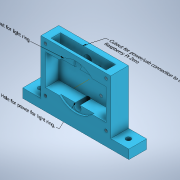
# Autodesk Inventor part: 2020PiZeroCameraLightRingMount
Saved by Autodesk Inventor 2020.2 (Build 242310000, 310)
## iProperties
Created: 2019-10-10
Part Number: 2020PiZeroCameraLightRingMount
Material: PC/ABS Plastic
Document SubType Name: Modeling
Designer: steele
Density: 0.357273 g/cm^3
Appearance: Turquoise
Author: steele
Autodesk Inventor part; units mm, degrees
ref_plane "YZ Plane" through (0, 0, 0) normal (1, 0, 0) x (0, 1, 0)
ref_plane "XZ Plane" through (0, 0, 0) normal (0, 1, 0) x (-1, 0, 0)
ref_plane "XY Plane" through (0, 0, 0) normal (0, 0, 1) x (1, 0, 0)
sketch "Sketch1" plane through (0, 0, 0) normal (0, 0, 1) x (1, 0, 0)
  line L0 (-48.5775, -37.85) -> (48.5775, -37.85)
  line L1 (48.5775, -37.85) -> (48.5775, 37.85)
  line L2 (48.5775, 37.85) -> (-48.5775, 37.85)
  line L3 (-48.5775, 37.85) -> (-48.5775, -37.85)
  line L4 (-48.5775, -37.85) -> (48.5775, 37.85) construction
  line L5 (48.5775, -37.85) -> (-48.5775, 37.85) construction
  point P0 (0, 0)
  dimension "majorPartWidth" = 97.155
  dimension "majorPartHeight" = 75.7
  constraints: 12 end point, 2 midpoint, 2 parallel, 1 horizontal, 1 perpendicular
  measures "majorPartWidth" distance of L0.start L0.end
  measures "majorPartHeight" distance of L1.end L0.end
extrude "Extrusion1" add sketch "Sketch1" against normal blind 24.725
sketch "Sketch2" plane through (0, 0, 0) normal (0, 0, 1) x (1, 0, 0)
  line L0 (-42.2275, -21.59) -> (42.2275, -21.59)
  line L1 (42.2275, -21.59) -> (42.2275, 21.59)
  line L2 (42.2275, 21.59) -> (-42.2275, 21.59)
  line L3 (-42.2275, 21.59) -> (-42.2275, -21.59)
  line L4 (-42.2275, -21.59) -> (42.2275, 21.59) construction
  line L5 (42.2275, -21.59) -> (-42.2275, 21.59) construction
  point P0 (0, 0)
  dimension "holeForPiCaseWidth" = 84.455
  dimension "holeForPiCaseHeight" = 43.18
  constraints: 12 end point, 2 midpoint, 2 parallel, 1 horizontal, 1 perpendicular
  measures "holeForPiCaseWidth" distance of L0.start L0.end
  measures "holeForPiCaseHeight" distance of L1.end L0.end
extrude "Extrusion2" cut sketch "Sketch2" against normal blind 18.375
sketch "Sketch3" plane through (0, 0, 0) normal (0, 0, 1) x (1, 0, 0)
  circle A0 centre (0, 0) radius 31.5
  circle A1 centre (0, 0) radius 18.5
  dimension "lightRingHoleExteriorDiam" = 63
  dimension "lightRingHoleInteriorDiam" = 37
  constraints: 2 centre point, 2 coincident
  measures "lightRingHoleExteriorDiam" diameter of A0
  measures "lightRingHoleInteriorDiam" diameter of A1
extrude "Extrusion3" cut sketch "Sketch3" against normal blind 2.5
sketch "Sketch4" plane through (0, 0, -2.5) normal (0, 0, 1) x (1, 0, 0)
  circle A0 centre (0, 0) radius 25.4466 construction
  circle A1 centre (0, 25.4466) radius 5
  circle A2 centre (0, -25.4466) radius 5
  dimension "holeForLightRingWires" = 10
  dimension "d13" = 10
  constraints: 3 centre point, 2 point on circle, 1 coincident
  measures "holeForLightRingWires" diameter of A1
  measures "d13" diameter of A2
extrude "Extrusion4" cut sketch "Sketch4" against normal through all
sketch "Sketch6" plane through (-48.5775, -37.85, 0) normal (0, -1, 0) x (1, 0, 0)
  line L0 (0, -24.725) -> (97.155, -24.725) projected
  line L1 (0, -24.725) -> (97.155, -24.725)
  line L2 (97.155, -24.725) -> (97.155, 0)
  line L3 (97.155, 0) -> (0, 0)
  line L4 (0, 0) -> (0, -24.725)
  point P0 (48.5775, 0)
  dimension "baseWidth" = 97.155
  dimension "baseDepth" = 24.725
  constraints: 8 end point, 2 parallel, 1 horizontal, 1 perpendicular
  measures "baseWidth" distance of L2.end L3.end
  measures "baseDepth" distance of L1.end L2.end
extrude "Extrusion6" add sketch "Sketch6" along normal blind 12.7
sketch "Sketch7" plane through (-48.5775, 37.85, 0) normal (0, 1, 0) x (1, 0, 0)
  line L0 (97.155, 0) -> (0, 0) construction
  line L1 (0, 0) -> (0, 24.725) construction
  line L2 (10.16, 3.77) -> (86.995, 3.77)
  line L3 (86.995, 3.77) -> (86.995, 17.105)
  line L4 (86.995, 17.105) -> (10.16, 17.105)
  line L5 (10.16, 17.105) -> (10.16, 3.77)
  line L6 (10.16, 3.77) -> (86.995, 17.105) construction
  line L7 (86.995, 3.77) -> (10.16, 17.105) construction
  line L8 (45.3952, 18.375) -> (45.3952, 2.5) projected
  point P0 (48.5775, 0)
  point P1 (48.5775, 10.4375)
  dimension "y" = 10.4375
  dimension "Y" = 48.5775
  dimension "piWireDepth" = 13.335
  dimension "piWireWidth" = 76.835
  constraints: 12 end point, 2 midpoint, 2 parallel, 2 perpendicular
  measures "y" distance from line of point (48.577, 10.438) L0
  measures "Y" distance from line of point (48.577, 10.438) L1
  measures "piWireDepth" distance of L4.end L2.start
  measures "piWireWidth" distance of L3.end L4.end
extrude "Extrusion7" cut sketch "Sketch7" against normal up to next
sketch "Sketch8" plane through (-48.5775, 37.85, -24.725) normal (-1, 0, 0) x (0, 0, 1)
  line L0 (24.725, -75.7) -> (24.725, 0) projected
  line L1 (24.725, -75.7) -> (28.535, -75.7)
  line L2 (28.535, -75.7) -> (28.535, -78.24)
  line L3 (28.535, -78.24) -> (24.725, -78.24)
  line L4 (24.725, -78.24) -> (24.725, -75.7)
  point P0 (24.725, -37.85)
  dimension "d30" = 3.81
  dimension "d31" = 2.54
  constraints: 8 end point, 2 parallel, 1 horizontal, 1 perpendicular
  measures "d30" distance of L2.end L3.end
  measures "d31" distance of L1.end L2.end
extrude "Extrusion8" cut sketch "Sketch8" against normal through all
sketch "Sketch9" plane through (0, 0, 0) normal (0, 0, 1) x (1, 0, 0)
  point P0 (-42.2275, 31.5)
  point P1 (42.2275, 31.5)
  point P2 (42.2275, -31.5)
  point P3 (-42.2275, -31.5)
hole "Hole1" at (-42.2275, 31.5, 0) at (42.2275, 31.5, 0) at (42.2275, -31.5, 0) at (-42.2275, -31.5, 0) direction (0, 0, -1) diameter 3.9624 depth 14.986 tip angle 120 thread size "10-32 UNF" class "2B" standard "ANSI Unified Screw Threads"
sketch "Sketch10" plane through (0, 0, -24.725) normal (0, 0, -1) x (-1, 0, 0)
  point P0 (-39.0525, 23.7022)
  point P1 (-16.8275, 23.7022)
  point P2 (-16.8275, -11.2228)
  point P3 (-39.0525, -11.2228)
hole "Hole3" at (39.0525, 23.7022, -24.725) at (16.8275, 23.7022, -24.725) at (16.8275, -11.2228, -24.725) at (39.0525, -11.2228, -24.725) direction (0, 0, 1) diameter 3.9624 depth 11.9507 tip angle 120 thread size "10-32 UNF" class "2B" standard "ANSI Unified Screw Threads"
sketch "Sketch14" plane through (-48.5775, -50.55, 0) normal (0, -1, 0) x (1, 0, 0)
  circle A0 centre (-12.7, 0) radius 2.5527 construction
  circle A1 centre (109.855, 0) radius 2.5527 construction
  line L0 (-12.7, 0) -> (109.855, 0) construction
  spline S0 degree 2 poles (34.1258, -3.8141) (34.1258, -4.5098) (33.5619, -5.6296) (33.0884, -5.9424) knots 0 0 0 1 2 2 2
  spline S1 degree 2 poles (33.0884, -5.9424) (32.7015, -6.1853) (31.9069, -6.35) (31.2894, -6.35) knots 0 0 0 1 2 2 2
  line L1 (31.2894, -6.35) -> (30.1203, -6.35)
  line L2 (30.1203, -6.35) -> (30.1203, -1.27)
  line L3 (30.1203, -1.27) -> (31.2771, -1.27)
  spline S2 degree 2 poles (31.2771, -1.27) (31.9934, -1.27) (32.8085, -1.4841) (33.0967, -1.6734) knots 0 0 0 1 2 2 2
  spline S3 degree 2 poles (33.0967, -1.6734) (33.5866, -1.9987) (34.1258, -3.0731) (34.1258, -3.8141) knots 0 0 0 1 2 2 2
  spline S4 degree 2 poles (33.4219, -3.8059) (33.4219, -3.2213) (33.0349, -2.3939) (32.6521, -2.1592) knots 0 0 0 1 2 2 2
  spline S5 degree 2 poles (32.6521, -2.1592) (32.3804, -1.9987) (31.767, -1.8546) (31.31, -1.8546) knots 0 0 0 1 2 2 2
  line L4 (31.31, -1.8546) -> (30.7954, -1.8546)
  line L5 (30.7954, -1.8546) -> (30.7954, -5.7654)
  line L6 (30.7954, -5.7654) -> (31.31, -5.7654)
  spline S6 degree 2 poles (31.31, -5.7654) (31.7587, -5.7654) (32.438, -5.6213) (32.7138, -5.4279) knots 0 0 0 1 2 2 2
  spline S7 degree 2 poles (32.7138, -5.4279) (33.0679, -5.1891) (33.4219, -4.3987) (33.4219, -3.8059) knots 0 0 0 1 2 2 2
  spline S8 degree 2 poles (36.4641, -6.4365) (35.5502, -6.4365) (34.5457, -5.4114) (34.5457, -4.4646) knots 0 0 0 1 2 2 2
  spline S9 degree 2 poles (34.5457, -4.4646) (34.5457, -3.5342) (35.5214, -2.4309) (36.3077, -2.4309) knots 0 0 0 1 2 2 2
  spline S10 degree 2 poles (36.3077, -2.4309) (36.6617, -2.4309) (37.2093, -2.6367) (37.411, -2.8549) knots 0 0 0 1 2 2 2
  spline S11 degree 2 poles (37.411, -2.8549) (37.6168, -3.0731) (37.835, -3.703) (37.835, -4.1599) knots 0 0 0 1 2 2 2
  line L7 (37.835, -4.1599) -> (37.835, -4.5098)
  line L8 (37.835, -4.5098) -> (35.1962, -4.5098)
  spline S12 degree 2 poles (35.1962, -4.5098) (35.1962, -5.1726) (35.8631, -5.8766) (36.4559, -5.8766) knots 0 0 0 1 2 2 2
  spline S13 degree 2 poles (36.4559, -5.8766) (36.6658, -5.8766) (37.0734, -5.7819) (37.2381, -5.7078) knots 0 0 0 1 2 2 2
  spline S14 degree 2 poles (37.2381, -5.7078) (37.411, -5.6255) (37.6497, -5.4814) (37.728, -5.4155) knots 0 0 0 1 2 2 2
  line L9 (37.728, -5.4155) -> (37.765, -5.4155)
  line L10 (37.765, -5.4155) -> (37.765, -6.1153)
  spline S15 degree 2 poles (37.765, -6.1153) (37.6539, -6.1606) (37.3163, -6.2924) (37.1846, -6.3294) knots 0 0 0 1 2 2 2
  spline S16 degree 2 poles (37.1846, -6.3294) (36.9993, -6.3829) (36.6947, -6.4365) (36.4641, -6.4365) knots 0 0 0 1 2 2 2
  spline S17 degree 2 poles (37.2093, -4.02) (37.201, -3.7606) (37.094, -3.3819) (36.9911, -3.2542) knots 0 0 0 1 2 2 2
  spline S18 degree 2 poles (36.9911, -3.2542) (36.8799, -3.1102) (36.53, -2.9578) (36.2706, -2.9578) knots 0 0 0 1 2 2 2
  spline S19 degree 2 poles (36.2706, -2.9578) (36.0154, -2.9578) (35.6573, -3.1102) (35.5091, -3.2584) knots 0 0 0 1 2 2 2
  spline S20 degree 2 poles (35.5091, -3.2584) (35.365, -3.4107) (35.2168, -3.7771) (35.1962, -4.02) knots 0 0 0 1 2 2 2
  line L11 (35.1962, -4.02) -> (37.2093, -4.02)
  spline S21 degree 2 poles (39.5146, -6.4406) (39.1317, -6.4406) (38.469, -6.2347) (38.2508, -6.1195) knots 0 0 0 1 2 2 2
  line L12 (38.2508, -6.1195) -> (38.2508, -5.399)
  line L13 (38.2508, -5.399) -> (38.2837, -5.399)
  spline S22 degree 2 poles (38.2837, -5.399) (38.366, -5.4649) (38.5883, -5.6213) (38.7736, -5.7078) knots 0 0 0 1 2 2 2
  spline S23 degree 2 poles (38.7736, -5.7078) (38.9341, -5.786) (39.3293, -5.9013) (39.5393, -5.9013) knots 0 0 0 1 2 2 2
  spline S24 degree 2 poles (39.5393, -5.9013) (39.6916, -5.9013) (40.0415, -5.8313) (40.1239, -5.7737) knots 0 0 0 1 2 2 2
  spline S25 degree 2 poles (40.1239, -5.7737) (40.2433, -5.6954) (40.3503, -5.5184) (40.3503, -5.3373) knots 0 0 0 1 2 2 2
  spline S26 degree 2 poles (40.3503, -5.3373) (40.3503, -5.1109) (40.1033, -4.8762) (39.7863, -4.798) knots 0 0 0 1 2 2 2
  spline S27 degree 2 poles (39.7863, -4.798) (39.6628, -4.7692) (39.2676, -4.6869) (39.0988, -4.6416) knots 0 0 0 1 2 2 2
  spline S28 degree 2 poles (39.0988, -4.6416) (38.6624, -4.514) (38.2672, -3.987) (38.2672, -3.6124) knots 0 0 0 1 2 2 2
  spline S29 degree 2 poles (38.2672, -3.6124) (38.2672, -3.0937) (39.0453, -2.4474) (39.6875, -2.4474) knots 0 0 0 1 2 2 2
  spline S30 degree 2 poles (39.6875, -2.4474) (40.0045, -2.4474) (40.6467, -2.6038) (40.8649, -2.7232) knots 0 0 0 1 2 2 2
  line L14 (40.8649, -2.7232) -> (40.8649, -3.4107)
  line L15 (40.8649, -3.4107) -> (40.8319, -3.4107)
  spline S31 degree 2 poles (40.8319, -3.4107) (40.5849, -3.2131) (39.9839, -2.9867) (39.6752, -2.9867) knots 0 0 0 1 2 2 2
  spline S32 degree 2 poles (39.6752, -2.9867) (39.3582, -2.9867) (38.9218, -3.2542) (38.9218, -3.5218) knots 0 0 0 1 2 2 2
  spline S33 degree 2 poles (38.9218, -3.5218) (38.9218, -3.7647) (39.1811, -3.9994) (39.4693, -4.0735) knots 0 0 0 1 2 2 2
  spline S34 degree 2 poles (39.4693, -4.0735) (39.6093, -4.1105) (39.9633, -4.1846) (40.1568, -4.2299) knots 0 0 0 1 2 2 2
  spline S35 degree 2 poles (40.1568, -4.2299) (40.5767, -4.3369) (41.0048, -4.8268) (41.0048, -5.2508) knots 0 0 0 1 2 2 2
  spline S36 degree 2 poles (41.0048, -5.2508) (41.0048, -5.4978) (40.8114, -5.9342) (40.622, -6.0948) knots 0 0 0 1 2 2 2
  spline S37 degree 2 poles (40.622, -6.0948) (40.4203, -6.2635) (39.9057, -6.4406) (39.5146, -6.4406) knots 0 0 0 1 2 2 2
  line L16 (42.2563, -6.35) -> (41.6141, -6.35)
  line L17 (41.6141, -6.35) -> (41.6141, -2.5379)
  line L18 (41.6141, -2.5379) -> (42.2563, -2.5379)
  line L19 (42.2563, -2.5379) -> (42.2563, -6.35)
  line L20 (42.3016, -1.904) -> (41.5729, -1.904)
  line L21 (41.5729, -1.904) -> (41.5729, -1.2371)
  line L22 (41.5729, -1.2371) -> (42.3016, -1.2371)
  line L23 (42.3016, -1.2371) -> (42.3016, -1.904)
  spline S38 degree 2 poles (43.3349, -6.9593) (43.4008, -6.9881) (43.6519, -7.0787) (43.8124, -7.1157) knots 0 0 0 1 2 2 2
  spline S39 degree 2 poles (43.8124, -7.1157) (43.9894, -7.161) (44.29, -7.2145) (44.467, -7.2145) knots 0 0 0 1 2 2 2
  spline S40 degree 2 poles (44.467, -7.2145) (44.7634, -7.2145) (45.1751, -7.0581) (45.2903, -6.9181) knots 0 0 0 1 2 2 2
  spline S41 degree 2 poles (45.2903, -6.9181) (45.4015, -6.7781) (45.4879, -6.4118) (45.4879, -6.1771) knots 0 0 0 1 2 2 2
  line L24 (45.4879, -6.1771) -> (45.4879, -5.8436)
  spline S42 degree 2 poles (45.4879, -5.8436) (45.2286, -6.0701) (44.7304, -6.2841) (44.3558, -6.2841) knots 0 0 0 1 2 2 2
  spline S43 degree 2 poles (44.3558, -6.2841) (43.7054, -6.2841) (42.9356, -5.3167) (42.9356, -4.4069) knots 0 0 0 1 2 2 2
  spline S44 degree 2 poles (42.9356, -4.4069) (42.9356, -3.9335) (43.2032, -3.2007) (43.4255, -2.9414) knots 0 0 0 1 2 2 2
  spline S45 degree 2 poles (43.4255, -2.9414) (43.6395, -2.6985) (44.2282, -2.4309) (44.5411, -2.4309) knots 0 0 0 1 2 2 2
  spline S46 degree 2 poles (44.5411, -2.4309) (44.8375, -2.4309) (45.2697, -2.5709) (45.4879, -2.6985) knots 0 0 0 1 2 2 2
  line L25 (45.4879, -2.6985) -> (45.525, -2.5379)
  line L26 (45.525, -2.5379) -> (46.1301, -2.5379)
  line L27 (46.1301, -2.5379) -> (46.1301, -5.9136)
  spline S47 degree 2 poles (46.1301, -5.9136) (46.1301, -6.8852) (45.2862, -7.7908) (44.4176, -7.7908) knots 0 0 0 1 2 2 2
  spline S48 degree 2 poles (44.4176, -7.7908) (44.1376, -7.7908) (43.5531, -7.7003) (43.302, -7.6262) knots 0 0 0 1 2 2 2
  line L28 (43.302, -7.6262) -> (43.302, -6.9593)
  line L29 (43.302, -6.9593) -> (43.3349, -6.9593)
  line L30 (45.4879, -5.3167) -> (45.4879, -3.2213)
  spline S49 degree 2 poles (45.4879, -3.2213) (45.2492, -3.106) (44.8457, -3.0072) (44.644, -3.0072) knots 0 0 0 1 2 2 2
  spline S50 degree 2 poles (44.644, -3.0072) (44.1582, -3.0072) (43.5984, -3.7235) (43.5984, -4.3946) knots 0 0 0 1 2 2 2
  spline S51 degree 2 poles (43.5984, -4.3946) (43.5984, -5.0285) (44.0224, -5.6913) (44.4999, -5.6913) knots 0 0 0 1 2 2 2
  spline S52 degree 2 poles (44.4999, -5.6913) (44.751, -5.6913) (45.278, -5.4937) (45.4879, -5.3167) knots 0 0 0 1 2 2 2
  line L31 (50.0533, -6.35) -> (49.4111, -6.35)
  line L32 (49.4111, -6.35) -> (49.4111, -4.1764)
  spline S53 degree 2 poles (49.4111, -4.1764) (49.4111, -3.9129) (49.3617, -3.4601) (49.2876, -3.3242) knots 0 0 0 1 2 2 2
  spline S54 degree 2 poles (49.2876, -3.3242) (49.2094, -3.1801) (48.9295, -3.0402) (48.6907, -3.0402) knots 0 0 0 1 2 2 2
  spline S55 degree 2 poles (48.6907, -3.0402) (48.4519, -3.0402) (47.9456, -3.2954) (47.7027, -3.5012) knots 0 0 0 1 2 2 2
  line L33 (47.7027, -3.5012) -> (47.7027, -6.35)
  line L34 (47.7027, -6.35) -> (47.0605, -6.35)
  line L35 (47.0605, -6.35) -> (47.0605, -2.5379)
  line L36 (47.0605, -2.5379) -> (47.7027, -2.5379)
  line L37 (47.7027, -2.5379) -> (47.7027, -2.962)
  spline S56 degree 2 poles (47.7027, -2.962) (47.9909, -2.7026) (48.5466, -2.4309) (48.8595, -2.4309) knots 0 0 0 1 2 2 2
  spline S57 degree 2 poles (48.8595, -2.4309) (49.4194, -2.4309) (50.0533, -3.1719) (50.0533, -3.8759) knots 0 0 0 1 2 2 2
  line L38 (50.0533, -3.8759) -> (50.0533, -6.35)
  spline S58 degree 2 poles (52.6098, -6.4365) (51.6959, -6.4365) (50.6914, -5.4114) (50.6914, -4.4646) knots 0 0 0 1 2 2 2
  spline S59 degree 2 poles (50.6914, -4.4646) (50.6914, -3.5342) (51.6671, -2.4309) (52.4534, -2.4309) knots 0 0 0 1 2 2 2
  spline S60 degree 2 poles (52.4534, -2.4309) (52.8074, -2.4309) (53.3549, -2.6367) (53.5566, -2.8549) knots 0 0 0 1 2 2 2
  spline S61 degree 2 poles (53.5566, -2.8549) (53.7625, -3.0731) (53.9807, -3.703) (53.9807, -4.1599) knots 0 0 0 1 2 2 2
  line L39 (53.9807, -4.1599) -> (53.9807, -4.5098)
  line L40 (53.9807, -4.5098) -> (51.3419, -4.5098)
  spline S62 degree 2 poles (51.3419, -4.5098) (51.3419, -5.1726) (52.0088, -5.8766) (52.6016, -5.8766) knots 0 0 0 1 2 2 2
  spline S63 degree 2 poles (52.6016, -5.8766) (52.8115, -5.8766) (53.2191, -5.7819) (53.3837, -5.7078) knots 0 0 0 1 2 2 2
  spline S64 degree 2 poles (53.3837, -5.7078) (53.5566, -5.6255) (53.7954, -5.4814) (53.8736, -5.4155) knots 0 0 0 1 2 2 2
  line L41 (53.8736, -5.4155) -> (53.9107, -5.4155)
  line L42 (53.9107, -5.4155) -> (53.9107, -6.1153)
  spline S65 degree 2 poles (53.9107, -6.1153) (53.7995, -6.1606) (53.462, -6.2924) (53.3302, -6.3294) knots 0 0 0 1 2 2 2
  spline S66 degree 2 poles (53.3302, -6.3294) (53.145, -6.3829) (52.8403, -6.4365) (52.6098, -6.4365) knots 0 0 0 1 2 2 2
  spline S67 degree 2 poles (53.3549, -4.02) (53.3467, -3.7606) (53.2397, -3.3819) (53.1367, -3.2542) knots 0 0 0 1 2 2 2
  spline S68 degree 2 poles (53.1367, -3.2542) (53.0256, -3.1102) (52.6757, -2.9578) (52.4163, -2.9578) knots 0 0 0 1 2 2 2
  spline S69 degree 2 poles (52.4163, -2.9578) (52.1611, -2.9578) (51.8029, -3.1102) (51.6547, -3.2584) knots 0 0 0 1 2 2 2
  spline S70 degree 2 poles (51.6547, -3.2584) (51.5106, -3.4107) (51.3624, -3.7771) (51.3419, -4.02) knots 0 0 0 1 2 2 2
  line L43 (51.3419, -4.02) -> (53.3549, -4.02)
  line L44 (57.5622, -6.35) -> (56.92, -6.35)
  line L45 (56.92, -6.35) -> (56.92, -5.963)
  spline S71 degree 2 poles (56.92, -5.963) (56.7718, -6.0865) (56.5536, -6.2512) (56.4054, -6.3212) knots 0 0 0 1 2 2 2
  spline S72 degree 2 poles (56.4054, -6.3212) (56.2695, -6.3871) (55.9773, -6.457) (55.7838, -6.457) knots 0 0 0 1 2 2 2
  spline S73 degree 2 poles (55.7838, -6.457) (55.4709, -6.457) (54.944, -6.1977) (54.7587, -5.9466) knots 0 0 0 1 2 2 2
  spline S74 degree 2 poles (54.7587, -5.9466) (54.5735, -5.6954) (54.3676, -4.9544) (54.3676, -4.4728) knots 0 0 0 1 2 2 2
  spline S75 degree 2 poles (54.3676, -4.4728) (54.3676, -3.9706) (54.627, -3.2378) (54.8534, -2.962) knots 0 0 0 1 2 2 2
  spline S76 degree 2 poles (54.8534, -2.962) (55.0634, -2.715) (55.652, -2.4309) (55.9773, -2.4309) knots 0 0 0 1 2 2 2
  spline S77 degree 2 poles (55.9773, -2.4309) (56.2613, -2.4309) (56.6853, -2.5585) (56.92, -2.6903) knots 0 0 0 1 2 2 2
  line L46 (56.92, -2.6903) -> (56.92, -1.0436)
  line L47 (56.92, -1.0436) -> (57.5622, -1.0436)
  line L48 (57.5622, -1.0436) -> (57.5622, -6.35)
  line L49 (56.92, -5.4237) -> (56.92, -3.2213)
  spline S78 degree 2 poles (56.92, -3.2213) (56.6812, -3.106) (56.3025, -3.0196) (56.0843, -3.0196) knots 0 0 0 1 2 2 2
  spline S79 degree 2 poles (56.0843, -3.0196) (55.5903, -3.0196) (55.0304, -3.7606) (55.0304, -4.4604) knots 0 0 0 1 2 2 2
  spline S80 degree 2 poles (55.0304, -4.4604) (55.0304, -5.1356) (55.4586, -5.8478) (55.932, -5.8478) knots 0 0 0 1 2 2 2
  spline S81 degree 2 poles (55.932, -5.8478) (56.1831, -5.8478) (56.6936, -5.6172) (56.92, -5.4237) knots 0 0 0 1 2 2 2
  spline S82 degree 2 poles (63.869, -4.3822) (63.869, -5.3167) (62.9633, -6.457) (62.2799, -6.457) knots 0 0 0 1 2 2 2
  spline S83 degree 2 poles (62.2799, -6.457) (61.9712, -6.457) (61.5307, -6.3047) (61.3166, -6.173) knots 0 0 0 1 2 2 2
  line L50 (61.3166, -6.173) -> (61.2754, -6.35)
  line L51 (61.2754, -6.35) -> (60.6744, -6.35)
  line L52 (60.6744, -6.35) -> (60.6744, -1.0436)
  line L53 (60.6744, -1.0436) -> (61.3166, -1.0436)
  line L54 (61.3166, -1.0436) -> (61.3166, -2.9373)
  spline S84 degree 2 poles (61.3166, -2.9373) (61.5595, -2.7191) (62.1235, -2.4309) (62.4816, -2.4309) knots 0 0 0 1 2 2 2
  spline S85 degree 2 poles (62.4816, -2.4309) (63.128, -2.4309) (63.869, -3.4642) (63.869, -4.3822) knots 0 0 0 1 2 2 2
  spline S86 degree 2 poles (63.2062, -4.4316) (63.2062, -3.7482) (62.7904, -3.0402) (62.3293, -3.0402) knots 0 0 0 1 2 2 2
  spline S87 degree 2 poles (62.3293, -3.0402) (62.07, -3.0402) (61.5348, -3.2872) (61.3166, -3.4765) knots 0 0 0 1 2 2 2
  line L55 (61.3166, -3.4765) -> (61.3166, -5.6625)
  spline S88 degree 2 poles (61.3166, -5.6625) (61.5595, -5.7819) (61.9341, -5.8807) (62.1564, -5.8807) knots 0 0 0 1 2 2 2
  spline S89 degree 2 poles (62.1564, -5.8807) (62.6463, -5.8807) (63.2062, -5.185) (63.2062, -4.4316) knots 0 0 0 1 2 2 2
  line L56 (67.5287, -2.5379) -> (65.4786, -7.7538)
  line L57 (65.4786, -7.7538) -> (64.7911, -7.7538)
  line L58 (64.7911, -7.7538) -> (65.4745, -6.1647)
  line L59 (65.4745, -6.1647) -> (64.0913, -2.5379)
  line L60 (64.0913, -2.5379) -> (64.7829, -2.5379)
  line L61 (64.7829, -2.5379) -> (65.8244, -5.362)
  line L62 (65.8244, -5.362) -> (66.8618, -2.5379)
  line L63 (66.8618, -2.5379) -> (67.5287, -2.5379)
  line L64 (36.5115, -14.8583) -> (35.6346, -14.8583)
  line L65 (35.6346, -14.8583) -> (34.0291, -12.837)
  line L66 (34.0291, -12.837) -> (33.2552, -12.837)
  line L67 (33.2552, -12.837) -> (33.2552, -14.8583)
  line L68 (33.2552, -14.8583) -> (32.58, -14.8583)
  line L69 (32.58, -14.8583) -> (32.58, -9.7783)
  line L70 (32.58, -9.7783) -> (33.8891, -9.7783)
  spline S90 degree 2 poles (33.8891, -9.7783) (34.3255, -9.7783) (34.9142, -9.873) (35.1818, -10.0459) knots 0 0 0 1 2 2 2
  spline S91 degree 2 poles (35.1818, -10.0459) (35.4494, -10.2188) (35.7581, -10.7581) (35.7581, -11.1574) knots 0 0 0 1 2 2 2
  spline S92 degree 2 poles (35.7581, -11.1574) (35.7581, -11.7131) (35.19, -12.4665) (34.7042, -12.6476) knots 0 0 0 1 2 2 2
  line L71 (34.7042, -12.6476) -> (36.5115, -14.8583)
  spline S93 degree 2 poles (35.0542, -11.2109) (35.0542, -10.9886) (34.8977, -10.6469) (34.7331, -10.5358) knots 0 0 0 1 2 2 2
  spline S94 degree 2 poles (34.7331, -10.5358) (34.589, -10.4411) (34.2061, -10.3629) (33.9262, -10.3629) knots 0 0 0 1 2 2 2
  line L72 (33.9262, -10.3629) -> (33.2552, -10.3629)
  line L73 (33.2552, -10.3629) -> (33.2552, -12.273)
  line L74 (33.2552, -12.273) -> (33.848, -12.273)
  spline S95 degree 2 poles (33.848, -12.273) (34.1403, -12.273) (34.6054, -12.1701) (34.766, -12.0095) knots 0 0 0 1 2 2 2
  spline S96 degree 2 poles (34.766, -12.0095) (34.9142, -11.8696) (35.0542, -11.4744) (35.0542, -11.2109) knots 0 0 0 1 2 2 2
  spline S97 degree 2 poles (39.9983, -12.9523) (39.9983, -13.9156) (39.0721, -14.9653) (38.2981, -14.9653) knots 0 0 0 1 2 2 2
  spline S98 degree 2 poles (38.2981, -14.9653) (37.5036, -14.9653) (36.5938, -13.8826) (36.5938, -12.9523) knots 0 0 0 1 2 2 2
  spline S99 degree 2 poles (36.5938, -12.9523) (36.5938, -11.9972) (37.5324, -10.9392) (38.2981, -10.9392) knots 0 0 0 1 2 2 2
  spline S100 degree 2 poles (38.2981, -10.9392) (39.0721, -10.9392) (39.9983, -11.9931) (39.9983, -12.9523) knots 0 0 0 1 2 2 2
  spline S101 degree 2 poles (39.3355, -12.9523) (39.3355, -12.2113) (38.7962, -11.4908) (38.2981, -11.4908) knots 0 0 0 1 2 2 2
  spline S102 degree 2 poles (38.2981, -11.4908) (37.8, -11.4908) (37.2566, -12.2113) (37.2566, -12.9523) knots 0 0 0 1 2 2 2
  spline S103 degree 2 poles (37.2566, -12.9523) (37.2566, -13.6727) (37.8, -14.4137) (38.2981, -14.4137) knots 0 0 0 1 2 2 2
  spline S104 degree 2 poles (38.2981, -14.4137) (38.7921, -14.4137) (39.3355, -13.685) (39.3355, -12.9523) knots 0 0 0 1 2 2 2
  spline S105 degree 2 poles (43.8515, -12.8905) (43.8515, -13.825) (42.9459, -14.9653) (42.2625, -14.9653) knots 0 0 0 1 2 2 2
  spline S106 degree 2 poles (42.2625, -14.9653) (41.9537, -14.9653) (41.5133, -14.813) (41.2992, -14.6813) knots 0 0 0 1 2 2 2
  line L75 (41.2992, -14.6813) -> (41.258, -14.8583)
  line L76 (41.258, -14.8583) -> (40.657, -14.8583)
  line L77 (40.657, -14.8583) -> (40.657, -9.5519)
  line L78 (40.657, -9.5519) -> (41.2992, -9.5519)
  line L79 (41.2992, -9.5519) -> (41.2992, -11.4455)
  spline S107 degree 2 poles (41.2992, -11.4455) (41.5421, -11.2274) (42.1061, -10.9392) (42.4642, -10.9392) knots 0 0 0 1 2 2 2
  spline S108 degree 2 poles (42.4642, -10.9392) (43.1105, -10.9392) (43.8515, -11.9725) (43.8515, -12.8905) knots 0 0 0 1 2 2 2
  spline S109 degree 2 poles (43.1887, -12.9399) (43.1887, -12.2565) (42.773, -11.5485) (42.3119, -11.5485) knots 0 0 0 1 2 2 2
  spline S110 degree 2 poles (42.3119, -11.5485) (42.0525, -11.5485) (41.5174, -11.7955) (41.2992, -11.9848) knots 0 0 0 1 2 2 2
  line L80 (41.2992, -11.9848) -> (41.2992, -14.1708)
  spline S111 degree 2 poles (41.2992, -14.1708) (41.5421, -14.2902) (41.9167, -14.389) (42.139, -14.389) knots 0 0 0 1 2 2 2
  spline S112 degree 2 poles (42.139, -14.389) (42.6289, -14.389) (43.1887, -13.6933) (43.1887, -12.9399) knots 0 0 0 1 2 2 2
  spline S113 degree 2 poles (48.1658, -14.9489) (47.6142, -14.9489) (46.8403, -14.7183) (46.4986, -14.5537) knots 0 0 0 1 2 2 2
  line L81 (46.4986, -14.5537) -> (46.4986, -13.7056)
  line L82 (46.4986, -13.7056) -> (46.548, -13.7056)
  spline S114 degree 2 poles (46.548, -13.7056) (46.8814, -14.0185) (47.7253, -14.3643) (48.1164, -14.3643) knots 0 0 0 1 2 2 2
  spline S115 degree 2 poles (48.1164, -14.3643) (48.6763, -14.3643) (49.2485, -13.8991) (49.2485, -13.5162) knots 0 0 0 1 2 2 2
  spline S116 degree 2 poles (49.2485, -13.5162) (49.2485, -13.2116) (48.948, -12.8329) (48.6228, -12.7382) knots 0 0 0 1 2 2 2
  spline S117 degree 2 poles (48.6228, -12.7382) (48.3881, -12.6723) (47.997, -12.5818) (47.7048, -12.5077) knots 0 0 0 1 2 2 2
  spline S118 degree 2 poles (47.7048, -12.5077) (47.4413, -12.4377) (47.0255, -12.2277) (46.865, -12.0589) knots 0 0 0 1 2 2 2
  spline S119 degree 2 poles (46.865, -12.0589) (46.7085, -11.8902) (46.5356, -11.4373) (46.5356, -11.1409) knots 0 0 0 1 2 2 2
  spline S120 degree 2 poles (46.5356, -11.1409) (46.5356, -10.5234) (47.4989, -9.6877) (48.244, -9.6877) knots 0 0 0 1 2 2 2
  spline S121 degree 2 poles (48.244, -9.6877) (48.6722, -9.6877) (49.4297, -9.8565) (49.7549, -10.0171) knots 0 0 0 1 2 2 2
  line L83 (49.7549, -10.0171) -> (49.7549, -10.8239)
  line L84 (49.7549, -10.8239) -> (49.7055, -10.8239)
  spline S122 degree 2 poles (49.7055, -10.8239) (49.4626, -10.6016) (48.7051, -10.2723) (48.2893, -10.2723) knots 0 0 0 1 2 2 2
  spline S123 degree 2 poles (48.2893, -10.2723) (47.82, -10.2723) (47.2396, -10.7128) (47.2396, -11.0709) knots 0 0 0 1 2 2 2
  spline S124 degree 2 poles (47.2396, -11.0709) (47.2396, -11.392) (47.5813, -11.7749) (47.9024, -11.8613) knots 0 0 0 1 2 2 2
  spline S125 degree 2 poles (47.9024, -11.8613) (48.1164, -11.919) (48.7381, -12.0672) (48.9439, -12.1289) knots 0 0 0 1 2 2 2
  spline S126 degree 2 poles (48.9439, -12.1289) (49.4667, -12.2895) (49.9525, -12.9358) (49.9525, -13.4092) knots 0 0 0 1 2 2 2
  spline S127 degree 2 poles (49.9525, -13.4092) (49.9525, -13.7097) (49.7096, -14.2861) (49.4914, -14.4878) knots 0 0 0 1 2 2 2
  spline S128 degree 2 poles (49.4914, -14.4878) (49.2485, -14.7101) (48.631, -14.9489) (48.1658, -14.9489) knots 0 0 0 1 2 2 2
  spline S129 degree 2 poles (51.7432, -14.9324) (51.2204, -14.9324) (50.6317, -14.3355) (50.6317, -13.6891) knots 0 0 0 1 2 2 2
  line L85 (50.6317, -13.6891) -> (50.6317, -11.5773)
  line L86 (50.6317, -11.5773) -> (50.1995, -11.5773)
  line L87 (50.1995, -11.5773) -> (50.1995, -11.0462)
  line L88 (50.1995, -11.0462) -> (50.6317, -11.0462)
  line L89 (50.6317, -11.0462) -> (50.6317, -9.9512)
  line L90 (50.6317, -9.9512) -> (51.2739, -9.9512)
  line L91 (51.2739, -9.9512) -> (51.2739, -11.0462)
  line L92 (51.2739, -11.0462) -> (52.4554, -11.0462)
  line L93 (52.4554, -11.0462) -> (52.4554, -11.5773)
  line L94 (52.4554, -11.5773) -> (51.2739, -11.5773)
  line L95 (51.2739, -11.5773) -> (51.2739, -13.3927)
  spline S130 degree 2 poles (51.2739, -13.3927) (51.2739, -13.6809) (51.2945, -13.9979) (51.3645, -14.1338) knots 0 0 0 1 2 2 2
  spline S131 degree 2 poles (51.3645, -14.1338) (51.4221, -14.2531) (51.6815, -14.3725) (51.9038, -14.3725) knots 0 0 0 1 2 2 2
  spline S132 degree 2 poles (51.9038, -14.3725) (52.0602, -14.3725) (52.3525, -14.2778) (52.4184, -14.249) knots 0 0 0 1 2 2 2
  line L96 (52.4184, -14.249) -> (52.4554, -14.249)
  line L97 (52.4554, -14.249) -> (52.4554, -14.8254)
  spline S133 degree 2 poles (52.4554, -14.8254) (52.2743, -14.8748) (51.9038, -14.9324) (51.7432, -14.9324) knots 0 0 0 1 2 2 2
  spline S134 degree 2 poles (54.5838, -14.9447) (53.6698, -14.9447) (52.6654, -13.9197) (52.6654, -12.9728) knots 0 0 0 1 2 2 2
  spline S135 degree 2 poles (52.6654, -12.9728) (52.6654, -12.0425) (53.641, -10.9392) (54.4273, -10.9392) knots 0 0 0 1 2 2 2
  spline S136 degree 2 poles (54.4273, -10.9392) (54.7814, -10.9392) (55.3289, -11.145) (55.5306, -11.3632) knots 0 0 0 1 2 2 2
  spline S137 degree 2 poles (55.5306, -11.3632) (55.7364, -11.5814) (55.9546, -12.2113) (55.9546, -12.6682) knots 0 0 0 1 2 2 2
  line L98 (55.9546, -12.6682) -> (55.9546, -13.0181)
  line L99 (55.9546, -13.0181) -> (53.3158, -13.0181)
  spline S138 degree 2 poles (53.3158, -13.0181) (53.3158, -13.6809) (53.9827, -14.3849) (54.5755, -14.3849) knots 0 0 0 1 2 2 2
  spline S139 degree 2 poles (54.5755, -14.3849) (54.7855, -14.3849) (55.193, -14.2902) (55.3577, -14.2161) knots 0 0 0 1 2 2 2
  spline S140 degree 2 poles (55.3577, -14.2161) (55.5306, -14.1338) (55.7694, -13.9897) (55.8476, -13.9238) knots 0 0 0 1 2 2 2
  line L100 (55.8476, -13.9238) -> (55.8846, -13.9238)
  line L101 (55.8846, -13.9238) -> (55.8846, -14.6236)
  spline S141 degree 2 poles (55.8846, -14.6236) (55.7735, -14.6689) (55.4359, -14.8007) (55.3042, -14.8377) knots 0 0 0 1 2 2 2
  spline S142 degree 2 poles (55.3042, -14.8377) (55.1189, -14.8912) (54.8143, -14.9447) (54.5838, -14.9447) knots 0 0 0 1 2 2 2
  spline S143 degree 2 poles (55.3289, -12.5282) (55.3206, -12.2689) (55.2136, -11.8902) (55.1107, -11.7625) knots 0 0 0 1 2 2 2
  spline S144 degree 2 poles (55.1107, -11.7625) (54.9995, -11.6185) (54.6496, -11.4661) (54.3903, -11.4661) knots 0 0 0 1 2 2 2
  spline S145 degree 2 poles (54.3903, -11.4661) (54.135, -11.4661) (53.7769, -11.6185) (53.6287, -11.7667) knots 0 0 0 1 2 2 2
  spline S146 degree 2 poles (53.6287, -11.7667) (53.4846, -11.919) (53.3364, -12.2854) (53.3158, -12.5282) knots 0 0 0 1 2 2 2
  line L102 (53.3158, -12.5282) -> (55.3289, -12.5282)
  spline S147 degree 2 poles (58.26, -14.9447) (57.3461, -14.9447) (56.3416, -13.9197) (56.3416, -12.9728) knots 0 0 0 1 2 2 2
  spline S148 degree 2 poles (56.3416, -12.9728) (56.3416, -12.0425) (57.3172, -10.9392) (58.1035, -10.9392) knots 0 0 0 1 2 2 2
  spline S149 degree 2 poles (58.1035, -10.9392) (58.4576, -10.9392) (59.0051, -11.145) (59.2068, -11.3632) knots 0 0 0 1 2 2 2
  spline S150 degree 2 poles (59.2068, -11.3632) (59.4126, -11.5814) (59.6308, -12.2113) (59.6308, -12.6682) knots 0 0 0 1 2 2 2
  line L103 (59.6308, -12.6682) -> (59.6308, -13.0181)
  line L104 (59.6308, -13.0181) -> (56.992, -13.0181)
  spline S151 degree 2 poles (56.992, -13.0181) (56.992, -13.6809) (57.6589, -14.3849) (58.2517, -14.3849) knots 0 0 0 1 2 2 2
  spline S152 degree 2 poles (58.2517, -14.3849) (58.4617, -14.3849) (58.8692, -14.2902) (59.0339, -14.2161) knots 0 0 0 1 2 2 2
  spline S153 degree 2 poles (59.0339, -14.2161) (59.2068, -14.1338) (59.4456, -13.9897) (59.5238, -13.9238) knots 0 0 0 1 2 2 2
  line L105 (59.5238, -13.9238) -> (59.5608, -13.9238)
  line L106 (59.5608, -13.9238) -> (59.5608, -14.6236)
  spline S154 degree 2 poles (59.5608, -14.6236) (59.4497, -14.6689) (59.1121, -14.8007) (58.9804, -14.8377) knots 0 0 0 1 2 2 2
  spline S155 degree 2 poles (58.9804, -14.8377) (58.7951, -14.8912) (58.4905, -14.9447) (58.26, -14.9447) knots 0 0 0 1 2 2 2
  spline S156 degree 2 poles (59.0051, -12.5282) (58.9969, -12.2689) (58.8898, -11.8902) (58.7869, -11.7625) knots 0 0 0 1 2 2 2
  spline S157 degree 2 poles (58.7869, -11.7625) (58.6757, -11.6185) (58.3258, -11.4661) (58.0665, -11.4661) knots 0 0 0 1 2 2 2
  spline S158 degree 2 poles (58.0665, -11.4661) (57.8112, -11.4661) (57.4531, -11.6185) (57.3049, -11.7667) knots 0 0 0 1 2 2 2
  spline S159 degree 2 poles (57.3049, -11.7667) (57.1608, -11.919) (57.0126, -12.2854) (56.992, -12.5282) knots 0 0 0 1 2 2 2
  line L107 (56.992, -12.5282) -> (59.0051, -12.5282)
  line L108 (60.9358, -14.8583) -> (60.2936, -14.8583)
  line L109 (60.2936, -14.8583) -> (60.2936, -9.5519)
  line L110 (60.2936, -9.5519) -> (60.9358, -9.5519)
  line L111 (60.9358, -9.5519) -> (60.9358, -14.8583)
  spline S160 degree 2 poles (63.5334, -14.9447) (62.6195, -14.9447) (61.6151, -13.9197) (61.6151, -12.9728) knots 0 0 0 1 2 2 2
  spline S161 degree 2 poles (61.6151, -12.9728) (61.6151, -12.0425) (62.5907, -10.9392) (63.377, -10.9392) knots 0 0 0 1 2 2 2
  spline S162 degree 2 poles (63.377, -10.9392) (63.731, -10.9392) (64.2786, -11.145) (64.4803, -11.3632) knots 0 0 0 1 2 2 2
  spline S163 degree 2 poles (64.4803, -11.3632) (64.6861, -11.5814) (64.9043, -12.2113) (64.9043, -12.6682) knots 0 0 0 1 2 2 2
  line L112 (64.9043, -12.6682) -> (64.9043, -13.0181)
  line L113 (64.9043, -13.0181) -> (62.2655, -13.0181)
  spline S164 degree 2 poles (62.2655, -13.0181) (62.2655, -13.6809) (62.9324, -14.3849) (63.5252, -14.3849) knots 0 0 0 1 2 2 2
  spline S165 degree 2 poles (63.5252, -14.3849) (63.7352, -14.3849) (64.1427, -14.2902) (64.3074, -14.2161) knots 0 0 0 1 2 2 2
  spline S166 degree 2 poles (64.3074, -14.2161) (64.4803, -14.1338) (64.7191, -13.9897) (64.7973, -13.9238) knots 0 0 0 1 2 2 2
  line L114 (64.7973, -13.9238) -> (64.8343, -13.9238)
  line L115 (64.8343, -13.9238) -> (64.8343, -14.6236)
  spline S167 degree 2 poles (64.8343, -14.6236) (64.7232, -14.6689) (64.3856, -14.8007) (64.2539, -14.8377) knots 0 0 0 1 2 2 2
  spline S168 degree 2 poles (64.2539, -14.8377) (64.0686, -14.8912) (63.764, -14.9447) (63.5334, -14.9447) knots 0 0 0 1 2 2 2
  spline S169 degree 2 poles (64.2786, -12.5282) (64.2703, -12.2689) (64.1633, -11.8902) (64.0604, -11.7625) knots 0 0 0 1 2 2 2
  spline S170 degree 2 poles (64.0604, -11.7625) (63.9492, -11.6185) (63.5993, -11.4661) (63.34, -11.4661) knots 0 0 0 1 2 2 2
  spline S171 degree 2 poles (63.34, -11.4661) (63.0847, -11.4661) (62.7266, -11.6185) (62.5784, -11.7667) knots 0 0 0 1 2 2 2
  spline S172 degree 2 poles (62.5784, -11.7667) (62.4343, -11.919) (62.2861, -12.2854) (62.2655, -12.5282) knots 0 0 0 1 2 2 2
  line L116 (62.2655, -12.5282) -> (64.2786, -12.5282)
  line L117 (46.8794, -18.1672) -> (45.1298, -23.2472)
  line L118 (45.1298, -23.2472) -> (44.4011, -23.2472)
  line L119 (44.4011, -23.2472) -> (42.6515, -18.1672)
  line L120 (42.6515, -18.1672) -> (43.3761, -18.1672)
  line L121 (43.3761, -18.1672) -> (44.784, -22.3868)
  line L122 (44.784, -22.3868) -> (46.1919, -18.1672)
  line L123 (46.1919, -18.1672) -> (46.8794, -18.1672)
  spline S173 degree 2 poles (50.4403, -20.7072) (50.4403, -22.0739) (49.6458, -23.3542) (48.8183, -23.3542) knots 0 0 0 1 2 2 2
  spline S174 degree 2 poles (48.8183, -23.3542) (47.9785, -23.3542) (47.1922, -22.0492) (47.1922, -20.7113) knots 0 0 0 1 2 2 2
  spline S175 degree 2 poles (47.1922, -20.7113) (47.1922, -19.3363) (47.9868, -18.0643) (48.8183, -18.0643) knots 0 0 0 1 2 2 2
  spline S176 degree 2 poles (48.8183, -18.0643) (49.654, -18.0643) (50.4403, -19.3816) (50.4403, -20.7072) knots 0 0 0 1 2 2 2
  spline S177 degree 2 poles (49.5676, -22.2551) (49.6664, -22.004) (49.7487, -21.23) (49.7487, -20.7072) knots 0 0 0 1 2 2 2
  spline S178 degree 2 poles (49.7487, -20.7072) (49.7487, -20.1844) (49.6664, -19.4146) (49.5634, -19.1552) knots 0 0 0 1 2 2 2
  spline S179 degree 2 poles (49.5634, -19.1552) (49.4605, -18.8958) (49.1024, -18.6283) (48.8183, -18.6283) knots 0 0 0 1 2 2 2
  spline S180 degree 2 poles (48.8183, -18.6283) (48.5343, -18.6283) (48.1679, -18.8958) (48.0609, -19.1634) knots 0 0 0 1 2 2 2
  spline S181 degree 2 poles (48.0609, -19.1634) (47.9579, -19.4228) (47.8838, -20.2132) (47.8838, -20.7113) knots 0 0 0 1 2 2 2
  spline S182 degree 2 poles (47.8838, -20.7113) (47.8838, -21.2465) (47.9497, -21.9628) (48.0567, -22.2427) knots 0 0 0 1 2 2 2
  spline S183 degree 2 poles (48.0567, -22.2427) (48.1555, -22.5062) (48.5219, -22.7902) (48.8183, -22.7902) knots 0 0 0 1 2 2 2
  spline S184 degree 2 poles (48.8183, -22.7902) (49.0983, -22.7902) (49.4646, -22.5227) (49.5676, -22.2551) knots 0 0 0 1 2 2 2
  spline S185 degree 2 poles (52.4616, -18.6488) (52.2763, -18.6488) (51.91, -18.7394) (51.7329, -18.8094) knots 0 0 0 1 2 2 2
  spline S186 degree 2 poles (51.7329, -18.8094) (51.5683, -18.8794) (51.3254, -19.0276) (51.2307, -19.0934) knots 0 0 0 1 2 2 2
  line L124 (51.2307, -19.0934) -> (51.1895, -19.0934)
  line L125 (51.1895, -19.0934) -> (51.1895, -18.373)
  spline S187 degree 2 poles (51.1895, -18.373) (51.4118, -18.2536) (52.1734, -18.0602) (52.5151, -18.0602) knots 0 0 0 1 2 2 2
  spline S188 degree 2 poles (52.5151, -18.0602) (52.8609, -18.0602) (53.3755, -18.2001) (53.5855, -18.3483) knots 0 0 0 1 2 2 2
  spline S189 degree 2 poles (53.5855, -18.3483) (53.8078, -18.5089) (54.0383, -18.9741) (54.0383, -19.2869) knots 0 0 0 1 2 2 2
  spline S190 degree 2 poles (54.0383, -19.2869) (54.0383, -19.7068) (53.4867, -20.3408) (53.0997, -20.4231) knots 0 0 0 1 2 2 2
  line L126 (53.0997, -20.4231) -> (53.0997, -20.4725)
  spline S191 degree 2 poles (53.0997, -20.4725) (53.2602, -20.5055) (53.6266, -20.6537) (53.7831, -20.8019) knots 0 0 0 1 2 2 2
  spline S192 degree 2 poles (53.7831, -20.8019) (53.9395, -20.946) (54.1371, -21.407) (54.1371, -21.7405) knots 0 0 0 1 2 2 2
  spline S193 degree 2 poles (54.1371, -21.7405) (54.1371, -22.0822) (53.9024, -22.6626) (53.6884, -22.8849) knots 0 0 0 1 2 2 2
  spline S194 degree 2 poles (53.6884, -22.8849) (53.4661, -23.1155) (52.8362, -23.3542) (52.4369, -23.3542) knots 0 0 0 1 2 2 2
  spline S195 degree 2 poles (52.4369, -23.3542) (52.054, -23.3542) (51.3048, -23.169) (51.0496, -23.0414) knots 0 0 0 1 2 2 2
  line L127 (51.0496, -23.0414) -> (51.0496, -22.3209)
  line L128 (51.0496, -22.3209) -> (51.099, -22.3209)
  spline S196 degree 2 poles (51.099, -22.3209) (51.313, -22.4774) (52.0376, -22.7655) (52.3957, -22.7655) knots 0 0 0 1 2 2 2
  spline S197 degree 2 poles (52.3957, -22.7655) (52.6057, -22.7655) (53.0256, -22.6338) (53.1656, -22.4815) knots 0 0 0 1 2 2 2
  spline S198 degree 2 poles (53.1656, -22.4815) (53.3014, -22.3292) (53.4455, -21.9669) (53.4455, -21.6911) knots 0 0 0 1 2 2 2
  spline S199 degree 2 poles (53.4455, -21.6911) (53.4455, -21.4153) (53.2849, -21.0571) (53.1409, -20.9542) knots 0 0 0 1 2 2 2
  spline S200 degree 2 poles (53.1409, -20.9542) (52.9968, -20.8513) (52.6057, -20.7731) (52.3751, -20.7731) knots 0 0 0 1 2 2 2
  line L129 (52.3751, -20.7731) -> (52.087, -20.7731)
  line L130 (52.087, -20.7731) -> (52.087, -20.2091)
  line L131 (52.087, -20.2091) -> (52.3134, -20.2091)
  spline S201 degree 2 poles (52.3134, -20.2091) (52.7704, -20.2091) (53.3467, -19.7727) (53.3467, -19.3569) knots 0 0 0 1 2 2 2
  spline S202 degree 2 poles (53.3467, -19.3569) (53.3467, -19.1634) (53.1985, -18.8876) (53.0791, -18.8053) knots 0 0 0 1 2 2 2
  spline S203 degree 2 poles (53.0791, -18.8053) (52.9515, -18.7188) (52.6386, -18.6488) (52.4616, -18.6488) knots 0 0 0 1 2 2 2
  point P0 (48.5775, 0)
  constraints: 2 end point, 2 horizontal
extrude "Extrusion11" cut sketch "Sketch14" against normal blind 3.175
sketch "Sketch15" plane through (48.5775, 37.85, 0) normal (1, 0, 0) x (0, 0, -1)
  line L0 (24.725, 0) -> (24.725, -88.4) projected
  line L1 (0, -88.4) -> (24.725, -88.4)
  line L2 (24.725, -88.4) -> (24.725, -75.7)
  line L3 (24.725, -75.7) -> (0, -75.7)
  line L4 (0, -75.7) -> (0, -88.4)
  point P0 (0, -37.85)
  dimension "d68" = 12.7
  constraints: 8 end point, 2 parallel, 1 horizontal, 1 perpendicular, 1 point on line
  measures "d68" distance of L2.end L1.end
extrude "Extrusion12" add sketch "Sketch15" along normal blind 25.4
sketch "Sketch16" plane through (48.5775, -37.85, 0) normal (0, 1, 0) x (1, 0, 0)
  line L0 (0, 24.725) -> (25.4, 24.725) projected
  line L1 (0, 0) -> (0, 24.725) projected
  point P0 (-48.5775, 0)
  point P1 (12.7, 12.025)
  dimension "d78" = 12.7
  dimension "d79" = 12.7
  measures "d78" distance from line of point (12.7, 12.025) L0
  measures "d79" distance from line of point (12.7, 12.025) L1
hole "Hole6" at (61.2775, -37.85, -12.025) direction (0, -1, 0) diameter 6.7564 end through all
mirror "Mirror2" about plane through (0, 0, 0) normal (1, 0, 0) of "Extrusion12", "Hole6"
equation "\"majorPartWidth\" = holeForPiCaseWidth + 2 * minWallThickness"
equation "\"majorPartHeight\" = lightRingHoleExteriorDiam + 2 * minWallThickness"
equation "\"majorPartDepth\" = holeForPiCaseDepth + minWallThickness"
equation "\"holeForPiCaseWidth\" = piCaseWidth + 2 * caseGap"
equation "\"holeForPiCaseHeight\" = piCaseHeight + 2 * caseGap"
equation "\"holeForPiCaseDepth\" = PiCaseDepth + depthForLightRing"
equation "\"lightRingHoleExteriorDiam\" = lightRingExteriorDiam + lightRingEdgeSpacing"
equation "\"lightRingHoleInteriorDiam\" = lightRingInterorDiam - lightRingEdgeSpacing"
equation "\"d13\" = holeForLightRingWires"
equation "\"baseWidth\" = majorPartWidth"
equation "\"baseDepth\" = majorPartDepth"
equation "\"y\" = 0.5 * PiCaseDepth + depthForLightRing"
equation "\"Y\" = 0.5 * majorPartWidth"
equation "\"minWallThickness\" = 6.35"
equation "\"lightRingEdgeSpacing\" = 3"
equation "\"lightRingExteriorDiam\" = 60"
equation "\"lightRingInterorDiam\" = 40"
equation "\"caseGap\" = 2.54"
equation "\"piCaseWidth\" = 79.375"
equation "\"piCaseHeight\" = 38.1"
equation "\"PiCaseDepth\" = 15.875"
equation "\"depthForLightRing\" = 2.5"
body "Solid1"
